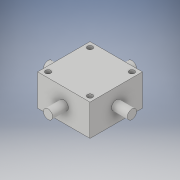
# Autodesk Inventor part: ZFSWHA-1-20+_Switch
Saved by Autodesk Inventor 2018 (Build 220112000, 112)
## iProperties
Created: 2018-04-10
Part Number: ZFSWHA-1-20+_Switch
Material: Generic
Document SubType Name: Modeling
Designer: bbramman
Density: 1 g/cm^3
Appearance: Default
Author: bbramman
Autodesk Inventor part; units mm, degrees
ref_plane "YZ Plane" through (0, 0, 0) normal (1, 0, 0) x (0, 1, 0)
ref_plane "XZ Plane" through (0, 0, 0) normal (0, 1, 0) x (-1, 0, 0)
ref_plane "XY Plane" through (0, 0, 0) normal (0, 0, 1) x (1, 0, 0)
sketch "Sketch1" plane through (0, 0, 0) normal (0, 1, 0) x (-1, 0, 0)
  line L0 (-15.875, -15.875) -> (15.875, -15.875)
  line L1 (15.875, -15.875) -> (15.875, 15.875)
  line L2 (15.875, 15.875) -> (-15.875, 15.875)
  line L3 (-15.875, 15.875) -> (-15.875, -15.875)
  line L4 (-15.875, -15.875) -> (15.875, 15.875) construction
  line L5 (15.875, -15.875) -> (-15.875, 15.875) construction
  point P0 (0, 0)
  dimension "d0" = 31.75
  dimension "d1" = 31.75
  constraints: 12 end point, 2 midpoint, 2 parallel, 1 horizontal, 1 perpendicular
  measures "d0" distance of L2.end L1.end
  measures "d1" distance of L1.end L0.end
extrude "Extrusion1" add sketch "Sketch1" along normal mid plane 19.05
sketch "Sketch2" plane through (0, 9.525, 0) normal (0, 1, 0) x (1, 0, 0)
  circle A0 centre (-12.7, -12.7) radius 1.5875
  circle A1 centre (-12.7, 12.7) radius 1.5875
  circle A2 centre (12.7, -12.7) radius 1.5875
  circle A3 centre (12.7, 12.7) radius 1.5875
  point P0 (0, 0)
  dimension "d4" = 3.175
  dimension "d5" = 3.175
  dimension "d6" = 3.175
  dimension "d7" = 3.175
  constraints: 4 centre point
  measures "d4" diameter of A0
  measures "d5" diameter of A1
  measures "d6" diameter of A2
  measures "d7" diameter of A3
extrude "Extrusion2" cut sketch "Sketch2" against normal through all
sketch "Sketch3" plane through (-15.875, 9.525, 15.875) normal (0, 0, 1) x (1, 0, 0)
  circle A0 centre (15.875, -9.525) radius 2.794
  dimension "d10" = 5.588
  constraints: 1 centre point, 1 coincident
  measures "d10" diameter of A0
sketch "Sketch4" plane through (15.875, -9.525, -15.875) normal (1, 0, 0) x (0, 0, -1)
  circle A0 centre (-15.875, 9.525) radius 2.794
  dimension "d11" = 5.588
  constraints: 1 centre point, 1 coincident
  measures "d11" diameter of A0
sketch "Sketch5" plane through (15.875, 9.525, -15.875) normal (0, 0, -1) x (-1, 0, 0)
  circle A0 centre (15.875, -9.525) radius 2.794
  dimension "d12" = 5.588
  constraints: 1 centre point, 1 coincident
  measures "d12" diameter of A0
sketch "Sketch6" plane through (-15.875, -9.525, 15.875) normal (-1, 0, 0) x (0, 0, 1)
  circle A0 centre (-15.875, 9.525) radius 2.794
  dimension "d13" = 5.588
  constraints: 1 centre point, 1 coincident
  measures "d13" diameter of A0
extrude "Extrusion3" add sketch "Sketch6" along normal blind 9.525
extrude "Extrusion4" add sketch "Sketch5" along normal blind 9.525
extrude "Extrusion5" add sketch "Sketch4" along normal blind 9.525
extrude "Extrusion6" add sketch "Sketch3" along normal blind 9.525
body "Solid1"
